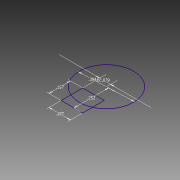
# Autodesk Inventor part: PG-Gearmotor-Shaft
Saved by Autodesk Inventor 2013 (Build 170138000, 138)
## iProperties
Created: 2013-01-27
Part Number: PG-Gearmotor-Shaft
Material: Aluminum 6061
Document SubType Name: Modeling
Designer: carneeki
Density: 1 g/cm^3
Author: carneeki
Autodesk Inventor part; units mm, degrees
ref_plane "YZ Plane" through (0, 0, 0) normal (1, 0, 0) x (0, 1, 0)
ref_plane "XZ Plane" through (0, 0, 0) normal (0, 1, 0) x (-1, 0, 0)
ref_plane "XY Plane" through (0, 0, 0) normal (0, 0, 1) x (1, 0, 0)
sketch "Sketch1" plane through (0, 0, 0) normal (0, 1, 0) x (-1, 0, 0)
  line L0 (-2, 7) -> (2, 7)
  line L1 (2, 7) -> (2, 4.5826)
  line L2 (-2, 4.5826) -> (-2, 7)
  line L3 (-5, 4.5826) -> (5, 4.5826) construction
  line L4 (0, 0) -> (5, 0)
  arc A0 (-2, 4.5826) -> (2, 4.5826) centre (0, 0) ccw
  dimension "d1" = 4
  dimension "d7" = 5
  dimension "d16" = 7
  dimension "d17" = 2.4174
  constraints: 10 end point, 2 parallel, 2 perpendicular, 2 point on circle, 2 point on line, 1 centre point, 1 coincident, 1 horizontal
  measures "d1" distance of L0.start L0.end
  measures "d7" radius of A0
  measures "d16" distance from line of L4.start L0
  measures "d17" distance between parallel lines of L3 L0
extrude "Extrusion1" add sketch "Sketch1" against normal blind 127
body "Solid1"
